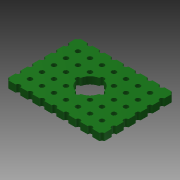
# Autodesk Inventor part: adapter
Saved by Autodesk Inventor 2013 (Build 170138000, 138)
## iProperties
Created: 2014-04-23
Part Number: adapter
Material: Generic
Document SubType Name: Modeling
Designer: Masta
Density: 1 g/cm^3
Author: Masta
Autodesk Inventor part; units mm, degrees
note: some values were not read from the file. Chosen so that the rebuilt part matches the saved one: copy form of "Rectangular Pattern1".
ref_plane "YZ Plane" through (0, 0, 0) normal (1, 0, 0) x (0, 1, 0)
ref_plane "XZ Plane" through (0, 0, 0) normal (0, 1, 0) x (-1, 0, 0)
ref_plane "XY Plane" through (0, 0, 0) normal (0, 0, 1) x (1, 0, 0)
sketch "Sketch1" plane through (0, 0, 0) normal (0, 0, 1) x (1, 0, 0)
  line L0 (10.16, -7.62) -> (-10.16, -7.62)
  line L1 (-10.16, -7.62) -> (-10.16, 7.62)
  line L2 (-10.16, 7.62) -> (10.16, 7.62)
  line L3 (10.16, 7.62) -> (10.16, -7.62)
  line L4 (10.16, -7.62) -> (-10.16, 7.62) construction
  line L5 (-10.16, -7.62) -> (10.16, 7.62) construction
  circle A0 centre (0, 0) radius 0.5
  circle A1 centre (0, 0) radius 2.5
  dimension "d0" = 20.32
  dimension "d1" = 15.24
  dimension "d17" = 1
  dimension "d20" = 5
  constraints: 12 end point, 4 midpoint, 2 centre point, 2 coincident, 2 parallel, 1 horizontal, 1 perpendicular
  measures "d0" distance of L1.end L2.end
  measures "d1" distance of L0.end L1.end
  measures "d17" diameter of A0
  measures "d20" diameter of A1
extrude "Extrusion1" add sketch "Sketch1" along normal blind 1.5 contours L0 L1 L2 L3 | A0 | A1
extrude "Extrusion2" cut sketch "Sketch1" along normal up to next contours A0
pattern_linear "Rectangular Pattern1" count 11 spacing 2.54 along (-1, 0, 0) count 7 spacing 2.54 along (0, -1, 0) of "Extrusion2" geometry pattern yes first direction both ways yes second direction both ways yes
extrude "Extrusion3" cut sketch "Sketch1" along normal up to next contours A0 | A1
body "Solid1"
